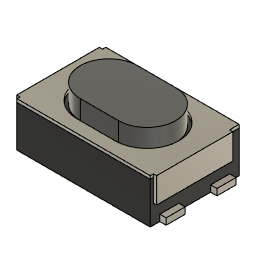
Tactile Microminiature 4.6x2.8x2.0mm v3 (Autodesk Fusion 360 design; units mm, degrees)
Autodesk Fusion 360 part; units mm, degrees
sketch "Sketch1" plane through (0, 0, 0) normal (0, 0, 1) x (1, 0, 0) in component "Tactile Microminiature CK KMR2"
  line L0 (-0.6, -1) -> (0.6, -1)
  arc A0 (0.6, -1) -> (0.6, 1) centre (0.6, 0) ccw
  line L1 (0.6, 1) -> (-0.6, 1)
  arc A1 (-0.6, 1) -> (-0.6, -1) centre (-0.6, 0) ccw
  line L2 (-0.6, 0) -> (0.6, 0) construction
  line L3 (0.6, 0.9) -> (-0.6, 0.9)
  arc A2 (-0.6, 0.9) -> (-0.6, -0.9) centre (-0.6, 0) ccw
  line L4 (-0.6, -0.9) -> (0.6, -0.9)
  arc A3 (0.6, -0.9) -> (0.6, 0.9) centre (0.6, 0) ccw
  line L5 (-2.2, 1.3) -> (-2.1, 1.3)
  line L6 (-2.1, -1.3) -> (-2.2, -1.3)
  line L7 (-2.2, -1.3) -> (-2.2, 1.3)
  line L8 (2.1, 1.3) -> (2.2, 1.3)
  line L9 (2.2, 1.3) -> (2.2, -1.3)
  line L10 (2.2, -1.3) -> (2.1, -1.3)
  line L11 (2.1, -1.4) -> (-2.1, -1.4)
  line L12 (-2.1, -1.4) -> (-2.1, 1.4)
  line L13 (-2.1, 1.4) -> (2.1, 1.4)
  line L14 (2.1, 1.4) -> (2.1, -1.4)
  line L15 (2.3, -0.5) -> (2.3, -1.1)
  line L16 (-2.3, -1.1) -> (-2.3, -0.5)
  line L17 (2.3, 1.1) -> (2.3, 0.5)
  line L18 (-2.3, 0.5) -> (-2.3, 1.1)
  line L19 (-2.3, 1.1) -> (-2.1, 1.1)
  line L20 (2.1, 1.1) -> (2.3, 1.1)
  line L21 (-2.1, 0.5) -> (-2.3, 0.5)
  line L22 (2.3, 0.5) -> (2.1, 0.5)
  line L23 (2.1, -0.5) -> (2.3, -0.5)
  line L24 (2.3, -1.1) -> (2.1, -1.1)
  line L25 (-2.1, -1.1) -> (-2.3, -1.1)
  line L26 (-2.3, -0.5) -> (-2.1, -0.5)
  dimension "d4" = -0.1
  dimension "d20" = 2.8
  constraint tangent L0 A0
  constraint tangent A0 L1
  constraint parallel L0 L1
  constraint tangent L1 A1
  constraint tangent L0 A1
  constraint horizontal L2
  constraint horizontal L5
  constraint horizontal L6
  constraint vertical L7
  constraint horizontal L8
  constraint vertical L9
  constraint horizontal L10
  constraint horizontal L13
  constraint vertical L14
  constraint horizontal L11
  constraint vertical L12
  constraint horizontal L26
  constraint vertical L15
  constraint horizontal L24
  constraint vertical L16
  constraint horizontal L19
  constraint vertical L17
  constraint horizontal L22
  constraint vertical L18
  constraint coincident L12 L19.end
  constraint coincident L14 L20.start
  constraint collinear L19 L20
  constraint coincident L12 L21.start
  constraint collinear L21 L22
  constraint coincident L14 L22.end
  constraint coincident L14 L23.start
  constraint collinear L23 L26
  constraint coincident L14 L24.end
  constraint coincident L12 L25.start
  constraint collinear L24 L25
  constraint coincident L12 L26.end
  measures "d20" distance of L12.end L11.end
extrude "Extrude2" add sketch "Sketch1" along normal blind 1.4 and the other way blind -1.3 contours L11 L12 L13 L14 makes body 1 in component "Tactile Microminiature CK KMR2"
extrude "Extrude3" add sketch "Sketch1" along normal blind 1.4 and the other way blind -0.6 contours L5 L7 L12 L19 | L7 L12 L19 L21 | L7 L12 L21 L26 | L7 L12 L25 L26 | L6 L7 L12 L25 | L9 L14 L20 L22 | L9 L14 L22 L23 | L9 L14 L23 L24 | L9 L10 L14 L24 bodies 1 in component "Tactile Microminiature CK KMR2"
extrude "Extrude4" add sketch "Sketch1" along normal blind 1.3 and the other way blind -1.9 separate body contours L3 A2 L4 A3 makes body 2 in component "Tactile Microminiature CK KMR2"
extrude "Extrude5" add sketch "Sketch1" along normal blind 1.3 separate body contours L0 A0 L1 A1 | L3 A2 L4 A3 | L11 L12 L13 L14 makes body 3 in component "Tactile Microminiature CK KMR2"
extrude "Extrude6" add sketch "Sketch1" along normal blind 0.2 separate body contours L7 L12 L19 L21 | L7 L18 L19 L21 | L7 L12 L25 L26 | L7 L16 L25 L26 | L9 L14 L20 L22 | L9 L17 L20 L22 | L9 L14 L23 L24 | L9 L15 L23 L24 makes body 4 at (-2.1667, 0.7, 0) makes body 5 at (2.1, 0.9, 0.0667) makes body 6 at (-2.1667, -0.9, 0) makes body 7 at (2.3, -0.7, 0.0667) in component "Tactile Microminiature CK KMR2"
component "Tactile Microminiature CK KMR2" placed x (1, 0, 0) y (0, 1, 0) z (0, 0, 1) at (0, 0, 0)
equation "d10 = 0.0 °"
equation "d14 = 0.0 °"
equation "d18 = 0.0 °"
